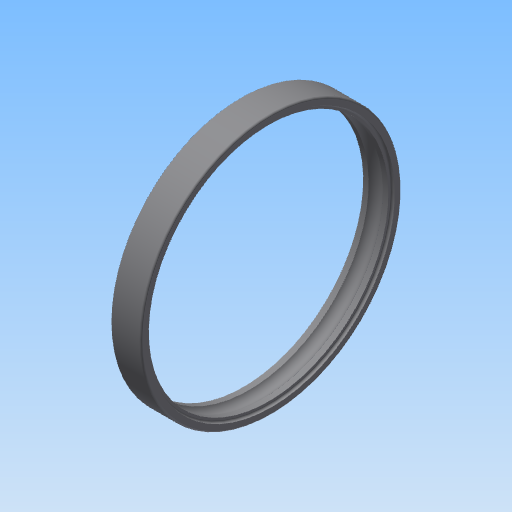
# Autodesk Inventor part: 61813-2RS1_PART2
Saved by Autodesk Inventor 2021 (Build 250183000, 183)
## iProperties
Category: PARTsolutions
Company: SKF
Created: 2020-03-01
Part Number: 61813-2RS1_PART2
Material: Allgemein
Catalog Web Link: www.cadenas.de
Description: -Deep groove ball bearings
Vendor: SKF
Document SubType Name: Modeling
Designer: psadmin
Manufacturer: SKF
Mass: 7.30918 g
Surface Area: 68.6748 cm^2
Volume: 7.30918 cm^3
Density: 1 g/cm^3
Appearance: PSOLRGB-175-175-175
PSOL_IDENT_0: {$CADENAS_DATA\23d-libs\skf\bearings_units_and_housings\ball_bearings\deep_groove_ball_bearings\bb1_
PSOL_IDENT_1: 001_101.prj},198 {VTYP=3D},{NB=61813-2RS1_PART2},{LINA=61813-2RS1_PART2},{NN=BB1_001_101_PART2},{NOP
PSOL_IDENT_2: RJ=TRUE},{DATE=19.12.2019 14:34:47},{GEOMDATE=18.12.2019 13:53:11},{VERSION=},{LINEID=7250},{WBVAR=}
PSOL_IDENT_3: ,{WBNUMERIC=}  {NB=61813-2RS1_PART2},{LINA=61813-2RS1_PART2},{KT=DUMMY},{PRODUCTID=1010271813},{DESI
PSOL_IDENT_4: GNATION=61813-2RS1},{DD=65.000},{D=85.000},{B=10.000},{C=0.000},{DD1=71.40},{DD2=0.00},{D1=0.00},{D2=
PSOL_IDENT_5: 80.50},{D3=0.000},{D4=0.000},{HH=MIN},{BB=0.000},{FF=0.00},{R0MAX=MIN},{R0=MIN},{R12=0.60},{PITCH=75
PSOL_IDENT_6: .00},{DW=5.556},{DDAMIN=68.200},{DDAMAX=71.500},{DDBMIN=MIN},{DDBMAX=MIN},{DBMIN=MIN},{DAMAX=81.800}
PSOL_IDENT_7: ,{BBAMIN=MIN},{CAMAX=MIN},{RAMAX=0.600},{LOAD1=12.400},{LOAD2=12.700},{LOAD3=0.540},{SPEED1=MIN},{SP
PSOL_IDENT_8: EED2=4500},{KR=0.015},{F0=17.000},{Z=23},{II=1},{MASS=0.130},{BEARING=61813-2RS1},{RING=},{HELP=3.13
PSOL_IDENT_9: 9},{HELP2=2.250},{DD1ALG=35.700},{YALG=35.700},{PITCH1=75.000},{DW1=5.556},{YALG1=39.361},{HALG1=3.1
PSOL_IDENT_10: 39},{SH=35.700},{CU=0.889},{DESIGN=dgbb2rs},{HALG=3.2},{B1=0},{SHIELDHELP=2}
NT: Deep groove ball bearings
NB: 61813-2RS1_PART2
NBSYN: $DESIGNATION._PART2
LINA: 61813-2RS1_PART2
SUPPLIER: SKF
ARTICLENO: 61813-2RS1_PART2
BOMINFO: 61813-2RS1_PART2
CREATOR: CADENAS GmbH
Title: 61813-2RS1_PART2
Author: Cadenas PARTsolutions
Comments: Deep groove ball bearings
Autodesk Inventor part; units mm, degrees
ref_plane "YZ Plane" through (0, 0, 0) normal (1, 0, 0) x (0, 1, 0)
ref_plane "XZ Plane" through (0, 0, 0) normal (0, 1, 0) x (-1, 0, 0)
ref_plane "XY Plane" through (0, 0, 0) normal (0, 0, 1) x (1, 0, 0)
sketch "Sketch_9" plane through (0, 0, 0) normal (0, 0, 1) x (1, 0, 0)
  line L0 (50, 0) -> (-50, 0)
  line L1 (0, 41.9) -> (0, 40.25)
  line L2 (0, 40.25) -> (0.3, 40.25)
  arc A0 (0.9, 39.65) -> (0.3, 40.25) centre (0.3, 39.65) ccw
  line L3 (0.9, 39.65) -> (0.9, 39.05)
  line L4 (0.9, 39.05) -> (2.6946, 39.05)
  arc A1 (7.3054, 39.05) -> (2.6946, 39.05) centre (5, 37.5) ccw
  line L5 (7.3054, 39.05) -> (9.1, 39.05)
  line L6 (9.1, 39.05) -> (9.1, 39.65)
  arc A2 (9.7, 40.25) -> (9.1, 39.65) centre (9.7, 39.65) ccw
  line L7 (9.7, 40.25) -> (10, 40.25)
  line L8 (10, 40.25) -> (10, 41.9)
  arc A3 (10, 41.9) -> (9.4, 42.5) centre (9.4, 41.9) ccw
  line L9 (9.4, 42.5) -> (0.6, 42.5)
  arc A4 (0.6, 42.5) -> (0, 41.9) centre (0.6, 41.9) ccw
  constraints: 20 end point, 10 point on circle, 5 centre point
revolve "Revolution1" add sketch "Sketch_9" angle 360 about axis through (50, 0, 0) along (1, 0, 0)
body "Solid1"
